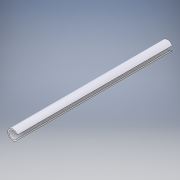
# Autodesk Inventor part: inner_sheath
Saved by Autodesk Inventor 2017 (Build 210142000, 142)
## iProperties
Created: 2018-11-30
Part Number: inner_sheath
Material: Acetal Resin, White
Document SubType Name: Modeling
Designer: ddeboer
Density: 1.425 g/cm^3
Appearance: Smooth - White
Author: ddeboer
Autodesk Inventor part; units mm, degrees
ref_plane "YZ Plane" through (0, 0, 0) normal (1, 0, 0) x (0, 1, 0)
ref_plane "XZ Plane" through (0, 0, 0) normal (0, 1, 0) x (-1, 0, 0)
sketch "Sketch1" plane through (0, 0, 0) normal (0, 0, 1) x (1, 0, 0)
  circle A0 centre (0, 0) radius 13.27
  circle A1 centre (0, 0) radius 10.325
  dimension "d0" = 26.54
  dimension "d1" = 20.65
  constraints: 2 centre point, 2 coincident
  measures "d0" diameter of A0
  measures "d1" diameter of A1
extrude "Extrusion1" add sketch "Sketch1" along normal blind 400
sketch "Sketch6" plane through (0, 0, 400) normal (0, 0, 1) x (1, 0, 0)
  line L0 (0, -5.75) -> (20, -5.75)
  line L1 (20, -5.75) -> (20, 5.75)
  line L2 (20, 5.75) -> (0, 5.75)
  line L3 (0, 5.75) -> (0, -5.75)
  point P0 (0, 0)
  point P1 (0, 0)
  dimension "d13" = 20
  dimension "d14" = 11.5
  constraints: 8 end point, 2 parallel, 1 coincident, 1 horizontal, 1 midpoint, 1 perpendicular
  measures "d13" distance of L2.end L1.end
  measures "d14" distance of L1.end L0.end
extrude "Extrusion5" cut sketch "Sketch6" against normal up to next
ref_plane "Work Plane2" through (11.9595, 5.75, 400) normal (1, 0, 0) x (0, -1, 0)
sketch "Sketch7" plane through (11.9595, 5.75, 400) normal (1, 0, 0) x (0, -1, 0)
  circle A0 centre (5.75, 375) radius 2
  line L0 (16.075, 0) -> (-4.575, 0) projected
  line L1 (-4.575, 400) -> (16.075, 400) projected
  point P0 (5.75, 400)
  point P1 (11.5, 0)
  point P2 (0, 0)
  point P3 (0, 400)
  point P4 (11.5, 400)
  dimension "d17" = 4
  dimension "d21" = 25
  constraints: 1 centre point
  measures "d17" diameter of A0
  measures "d21" distance from line of A0.centre L1
extrude "Extrusion6" cut sketch "Sketch7" against normal through all
body "Solid1"
